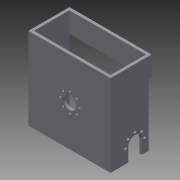
# Autodesk Inventor part: Arm_Bracket
Saved by Autodesk Inventor 2013 (Build 170138000, 138)
## iProperties
Created: 2014-04-11
Part Number: Arm_Bracket
Material: 一般
Document SubType Name: Modeling
Designer: andou
Density: 1 g/cm^3
Author: andou
Autodesk Inventor part; units mm, degrees
ref_plane "YZ Plane" through (0, 0, 0) normal (1, 0, 0) x (0, 1, 0)
ref_plane "XZ Plane" through (0, 0, 0) normal (0, 1, 0) x (-1, 0, 0)
ref_plane "XY Plane" through (0, 0, 0) normal (0, 0, 1) x (1, 0, 0)
sketch "スケッチ1" plane through (0, 0, 0) normal (0, 0, 1) x (1, 0, 0)
  line L0 (-30, 15) -> (30, 15)
  line L1 (30, 15) -> (30, -15)
  line L2 (30, -15) -> (-30, -15)
  line L3 (-30, -15) -> (-30, 15)
  line L4 (-28, 13) -> (28, 13)
  line L5 (28, 13) -> (28, -13)
  line L6 (28, -13) -> (-28, -13)
  line L7 (-28, -13) -> (-28, 13)
  point P0 (0, 0)
  dimension "d0" = 60
  dimension "d2" = 2
  dimension "d3" = 2
  dimension "d4" = 30
  dimension "d5" = 15
  dimension "d6" = 30
  dimension "d7" = 56
  dimension "d8" = 26
  constraints: 16 end point, 4 parallel, 2 horizontal, 2 perpendicular
  measures "d0" distance of L0.start L0.end
  measures "d2" distance between parallel lines of L1 L5
  measures "d3" distance between parallel lines of L2 L6
  measures "d4" distance from line of point (0, 0) L3
  measures "d5" distance from line of L0 point (0, 0)
  measures "d6" distance of L2.end L0.start
  measures "d7" distance between parallel lines of L5 L7
  measures "d8" distance between parallel lines of L6 L4
extrude "押し出し1" add sketch "スケッチ1" against normal blind 60
sketch "スケッチ2" plane through (-30, 15, 0) normal (0, 1, 0) x (1, 0, 0)
  line L0 (0, 0) -> (60, 0) projected
  line L1 (60, 0) -> (60, 60) projected
  line L2 (0, 60) -> (60, 60)
  line L3 (60, 60) -> (60, 15)
  line L4 (60, 15) -> (0, 15)
  line L5 (0, 15) -> (0, 60)
  point P0 (30, 0)
  dimension "d11" = 15
  constraints: 8 end point, 2 parallel, 1 horizontal, 1 perpendicular, 1 point on line
  measures "d11" distance between parallel lines of L0 L4
extrude "押し出し2" cut sketch "スケッチ2" against normal blind 2
sketch "スケッチ3" plane through (30, -15, 0) normal (1, 0, 0) x (0, 0, -1)
  line L0 (0, 0) -> (60, 0) projected
  line L1 (60, 28) -> (60, 0) projected
  arc A0 (50, 22) -> (50, 14) centre (50, 18) ccw
  line L2 (50, 22) -> (60, 22)
  line L3 (50, 14) -> (60, 14)
  point P0 (0, 15)
  dimension "d14" = 8
  dimension "d16" = 10
  dimension "d17" = 18
  constraints: 4 end point, 2 point on circle, 2 tangent, 1 centre point, 1 midpoint, 1 parallel, 1 perpendicular, 1 point on line
  measures "d14" diameter of A0
  measures "d16" distance from line of L1 A0.centre
  measures "d17" distance from line of L0 A0.centre
extrude "押し出し3" cut sketch "スケッチ3" against normal blind 60
sketch "スケッチ4" plane through (30, -15, 0) normal (1, 0, 0) x (0, 0, -1)
  line L0 (50, 22) -> (60, 22) projected
  line L1 (60, 28) -> (60, 22) projected
  line L2 (60, 14) -> (60, 0) projected
  line L3 (60, 14) -> (50, 14) projected
  arc A0 (50, 22) -> (50, 14) centre (50, 18) ccw projected
  arc A1 (50, 23) -> (50, 13) centre (50, 18) ccw
  line L4 (50, 23) -> (60, 23)
  line L5 (50, 13) -> (60, 13)
  point P0 (0, 15)
  dimension "d20" = 10
  constraints: 4 end point, 2 point on circle, 2 point on line, 2 tangent, 1 centre point, 1 coincident, 1 parallel, 1 perpendicular
  measures "d20" diameter of A1
extrude "押し出し4" cut sketch "スケッチ4" against normal blind 2
sketch "スケッチ5" plane through (30, -15, 0) normal (1, 0, 0) x (0, 0, -1)
  line L0 (60, 28) -> (60, 23) projected
  arc A0 (50, 23) -> (50, 13) centre (50, 18) ccw projected
  circle A1 centre (50, 25) radius 1
  point P0 (0, 15)
  dimension "d24" = 2
  dimension "d26" = 7
  dimension "d27" = 10
  constraints: 1 centre point
  measures "d24" diameter of A1
  measures "d26" distance of A1.centre A0.centre
  measures "d27" distance from line of L0 A1.centre
hole "穴1" at (30, 10, -50) direction (-1, 0, 0) diameter 2 end through all
pattern_circular "円形状パターン1" count 5 over 180 about axis through (30, 3, -50) along (1, 0, 0) of "穴1"
sketch "スケッチ6" plane through (-30, -15, 0) normal (0, -1, 0) x (1, 0, 0)
  line L0 (60, 0) -> (0, 0) projected
  line L1 (0, 0) -> (0, -60) projected
  circle A0 centre (30, -30) radius 5
  point P0 (30, 0)
  dimension "d38" = 10
  dimension "d40" = 30
  dimension "d41" = 30
  constraints: 1 centre point
  measures "d38" diameter of A0
  measures "d40" distance from line of L0 A0.centre
  measures "d41" distance from line of A0.centre L1
hole "穴2" at (0, -15, -30) direction (0, 1, 0) diameter 10 end through all
sketch "スケッチ7" plane through (-30, -15, 0) normal (0, -1, 0) x (1, 0, 0)
  circle A0 centre (30, -30) radius 5 projected
  line L0 (60, 0) -> (60, -60) projected
  circle A1 centre (30, -23) radius 1
  point P0 (30, 0)
  dimension "d49" = 2
  dimension "d51" = 7
  dimension "d52" = 30
  constraints: 1 centre point
  measures "d49" diameter of A1
  measures "d51" distance of A0.centre A1.centre
  measures "d52" distance from line of L0 A1.centre
hole "穴3" at (0, -15, -23) direction (0, 1, 0) diameter 2 depth 2 tip angle 118
pattern_circular "円形状パターン2" count 8 over 360 about axis through (0, 75, -30) along (0, -1, 0) of "穴3"
